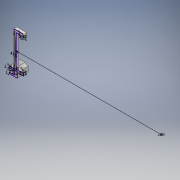
# Autodesk Inventor part: LeftClip
Saved by Autodesk Inventor 2017 (Build 210142000, 142)
## iProperties
Created: 2017-12-02
Part Number: LeftClip
Material: Generic
Document SubType Name: Modeling
Designer: Max
Density: 1 g/cm^3
Appearance: Default
Author: Max
Autodesk Inventor part; units mm, degrees
ref_plane "YZ Plane" through (0, 0, 0) normal (1, 0, 0) x (0, 1, 0)
ref_plane "XZ Plane" through (0, 0, 0) normal (0, 1, 0) x (-1, 0, 0)
ref_plane "XY Plane" through (0, 0, 0) normal (0, 0, 1) x (1, 0, 0)
sketch "Sketch1" plane through (0, 0, 0) normal (0, 1, 0) x (-1, 0, 0)
  line L0 (10.2, -3) -> (10.2, -46.7)
  line L1 (10.2, -46.7) -> (0.5, -46.7)
  line L2 (0.5, -46.7) -> (0.5, -45.95)
  line L3 (0.5, -45.95) -> (0, -45.95)
  line L4 (0, -45.95) -> (0, -46.7)
  line L5 (0.5, -3) -> (0.5, -3.75)
  line L6 (0.5, -3.75) -> (0, -3.75)
  line L7 (0, -3.75) -> (0, -3)
  line L8 (0, -3) -> (0, 0)
  line L9 (0, 0) -> (13.2, 0)
  line L10 (13.2, 0) -> (13.2, -47.45)
  line L11 (0, -49.7) -> (0, -46.7)
  line L12 (10.2, -3) -> (0.5, -3)
  line L13 (8.7, -56.4) -> (19.7, -56.4)
  line L14 (19.7, -56.4) -> (19.7, -54.7)
  line L15 (19.7, -54.7) -> (12.7, -54.7)
  line L16 (12.7, -54.7) -> (12.7, -49.7)
  line L17 (12.7, -49.7) -> (13.2, -49.7)
  line L18 (19.7, -49.7) -> (19.7, -47.45)
  line L19 (19.7, -47.45) -> (13.2, -47.45)
  line L20 (8.7, -56.4) -> (8.7, -49.7)
  arc A0 (10.2, -46.7) -> (10.2, -3) centre (-188.6029, -24.85) ccw
  line L21 (13.2, -49.7) -> (19.7, -49.7)
  line L22 (12.7, -49.7) -> (12.7, -49.7)
  line L23 (8.7, -49.7) -> (0, -49.7)
  line L24 (13.2, -47.45) -> (8.7, -49.7)
  point P0 (0, 0)
  dimension "d1" = 9.7
  dimension "d2" = 0.75
  dimension "d3" = 0.5
  dimension "d6" = 0.5
  dimension "d10" = 43.7
  dimension "d11" = 3
  dimension "d13" = 0.75
  dimension "d14" = 3
  dimension "d16" = 5
  dimension "d19" = 7
  dimension "d25" = 200
  dimension "d30" = 2.25
  dimension "d31" = 1.7
  dimension "d33" = 4.5
  dimension "d34" = 2.25
  dimension "d37" = 4
  constraints: 50 end point, 21 perpendicular, 5 point on line, 2 equal length, 2 horizontal, 2 point on circle, 1 centre point, 1 coincident
  measures "d1" distance of L0.end L1.end
  measures "d2" distance of L1.end L2.end
  measures "d3" distance of L2.end L3.end
  measures "d6" distance of L5.end L6.end
  measures "d10" distance of L0.start L0.end
  measures "d11" distance between parallel lines of L10 L0
  measures "d13" distance between parallel lines of L6 L12
  measures "d14" distance between parallel lines of L9 L12
  measures "d16" distance of L15.end L17.start
  measures "d19" distance of L17.start L18.start
  measures "d25" radius of A0
  measures "d30" distance of L18.start L18.end
  measures "d31" distance of L13.end L14.end
  measures "d33" distance from line of L20.end L10
  measures "d34" distance from line of L23 L10.end
  measures "d37" distance between parallel lines of L20 L16
extrude "Extrusion4" add sketch "Sketch1" along normal blind 4 contours L12 L5 L6 L7 L8 L9 L10 L24 L23 L11 L4 L3 L2 L1 A0
extrude "Extrusion5" add sketch "Sketch1" along normal blind 15 contours L24 L19 L18 L21 L17 L16 L15 L14 L13 L20
body "Solid1"
